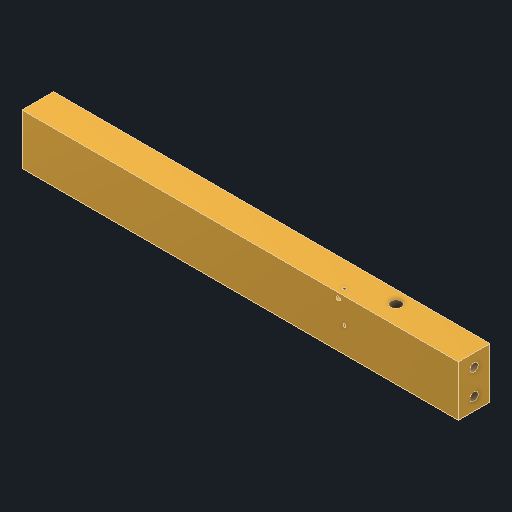
# Autodesk Inventor part: Main Piller
Saved by Autodesk Inventor 2027.1 (Build 311270010, 270A)
## iProperties
Created: 2025-09-16
Material: Brass, Soft Yellow
Document SubType Name: Modeling
Designer: SD
Density: 8.47 g/cm^3
Appearance: Brass - Satin
Mass: 2727.37 g
Surface Area: 492.65 cm^2
Volume: 340.921 cm^3
Project: Automatic Tea Steeping mechanism
Part Number: Main Piller
Thickness: 25.000 mm
Length: 345.000 mm
Width: 40.000 mm
BOM-Mass: 2.72737
BOM-Area: 0.049
Procurement: Fabricate - 1st round
Build Stage: 1
Preferred Material: C36000 Brass
Author: SD
Title: Main Piller
Autodesk Inventor part; units mm, degrees
ref_plane "YZ Plane" through (0, 0, 0) normal (1, 0, 0) x (0, 1, 0)
ref_plane "XZ Plane" through (0, 0, 0) normal (0, 1, 0) x (-1, 0, 0)
ref_plane "XY Plane" through (0, 0, 0) normal (0, 0, 1) x (1, 0, 0)
sketch "Sketch1" plane through (0, 0, 0) normal (1, 0, 0) x (0, 1, 0)
  line L0 (-20, 12.5) -> (20, 12.5)
  line L1 (20, 12.5) -> (20, -12.5)
  line L2 (20, -12.5) -> (-20, -12.5)
  line L3 (-20, -12.5) -> (-20, 12.5)
  line L4 (-20, 12.5) -> (20, -12.5) construction
  line L5 (20, 12.5) -> (-20, -12.5) construction
  point P0 (0, 0)
  dimension "Width" = 40
  dimension "Thickness" = 25
  constraints: 12 end point, 2 midpoint, 2 parallel, 1 horizontal, 1 perpendicular
  measures "Width" distance of L1.end L2.end
  measures "Thickness" distance of L0.end L1.end
extrude "Extrusion1" add sketch "Sketch1" along normal mid plane 345
sketch "Sketch2" plane through (-172.5, 0, 0) normal (-1, 0, 0) x (0, 0, 1)
  point P0 (0, 0)
  point P1 (0, 10)
  point P2 (0, -10)
  dimension "d4" = 20
  dimension "d5" = 10
  constraints: 2 vertical alignment
  measures "d4" distance of point (0, -10) point (0, 10)
  measures "d5" distance of point (0, 0) point (0, 10)
hole "Hole1" at (-172.5, 10, 0) at (-172.5, -10, 0) direction (1, 0, 0) diameter 4.917 depth 20 tip angle 118 thread size "M6x1" class "6H" standard "ISO Metric profile"
sketch "Sketch3" plane through (-172.5, 20, 12.5) normal (0, 1, 0) x (1, 0, 0)
  line L0 (345, 25) -> (345, 0) projected
  line L1 (0, 25) -> (345, 25) projected
  point P0 (172.5, 12.5)
  point P1 (280.7116, 15)
  dimension "d13" = 64.2884
  dimension "d14" = 10
  measures "d13" distance from line of point (280.712, 15) L0
  measures "d14" distance from line of point (280.712, 15) L1
hole "Hole2" at (108.2116, 20, -2.5) direction (0, -1, 0) diameter 8.376 depth 15 tip angle 118 thread size "M10x1.5" class "6H" standard "ISO Metric profile"
sketch "Sketch4" plane through (172.5, 20, -12.5) normal (0, 0, -1) x (-1, 0, 0)
  line L0 (345, 0) -> (345, -40) projected
  line L1 (0, -40) -> (345, -40) projected
  point P0 (172.5, -20)
  point P1 (325, -20)
  dimension "d22" = 20
  dimension "d23" = 20
  measures "d22" distance from line of point (325, -20) L0
  measures "d23" distance from line of point (325, -20) L1
hole "Hole3" at (-152.5, 0, -12.5) direction (0, 0, 1) diameter 8.376 depth 20 tip angle 118 thread size "M10x1.5" class "6H" standard "ISO Metric profile"
sketch "Sketch5" plane through (172.5, 0, 0) normal (1, 0, 0) x (0, 0, -1)
  circle A0 centre (0, 10) radius 2.4585 projected
  circle A1 centre (0, -10) radius 2.4585 projected
  point P0 (0, 0)
  constraints: 2 coincident
hole "Hole4" at (172.5, 10, 0) at (172.5, -10, 0) direction (-1, 0, 0) diameter 6.647 depth 16 tip angle 118 thread size "M8x1.25" class "6H" standard "ISO Metric profile"
sketch "Sketch6" plane through (-172.5, -20, 12.5) normal (0, 0, 1) x (1, 0, 0)
  line L0 (345, 40) -> (345, 0) projected
  point P0 (172.5, 20)
  point P1 (255, 20)
  dimension "d38" = 90
  constraints: 1 horizontal alignment
  measures "d38" distance from line of L0 point (255, 20)
hole "Hole5" at (82.5, 0, 12.5) direction (0, 0, -1) diameter 2.459 depth 10 tip angle 118 thread size "M3x0.5" class "6H" standard "ISO Metric profile"
sketch "Sketch7" plane through (-172.5, -20, 12.5) normal (0, 0, 1) x (1, 0, 0)
  line L0 (345, 40) -> (345, 0) projected
  line L1 (0, 40) -> (345, 40) projected
  point P0 (172.5, 20)
  point P1 (250, 36)
  dimension "d46" = 95
  dimension "d47" = 4
  measures "d46" distance from line of L0 point (250, 36)
  measures "d47" distance from line of L1 point (250, 36)
hole "Hole6" at (77.5, 16, 12.5) direction (0, 0, -1) diameter 3 depth 8
sketch "Sketch9" plane through (-172.5, -20, 12.5) normal (0, 0, 1) x (1, 0, 0)
  line L0 (251.5, 34.5) -> (248.5, 34.5)
  line L1 (248.5, 34.5) -> (248.5, 37.5)
  line L2 (248.5, 37.5) -> (251.5, 37.5)
  line L3 (251.5, 37.5) -> (251.5, 34.5)
  line L4 (251.5, 34.5) -> (248.5, 37.5) construction
  line L5 (248.5, 34.5) -> (251.5, 37.5) construction
  line L6 (0, 40) -> (345, 40) projected
  line L7 (345, 40) -> (345, 0) projected
  point P0 (250, 36)
  dimension "d67" = 4
  dimension "d68" = 95
  dimension "d69" = 3
  constraints: 12 end point, 2 midpoint, 2 parallel, 2 perpendicular, 1 horizontal
  measures "d67" distance from line of point (250, 36) L6
  measures "d68" distance from line of L7 point (250, 36)
  measures "d69" distance of L0.start L0.end
extrude "Extrusion2" [suppressed]
sketch "Sketch8" plane through (-172.5, 20, 12.5) normal (0, 1, 0) x (1, 0, 0)
  line L0 (345, 25) -> (345, 0) projected
  line L1 (0, 0) -> (345, 0) projected
  point P0 (172.5, 12.5)
  point P1 (250, 5)
  dimension "d55" = 95
  dimension "d56" = 5
  measures "d55" distance from line of L0 point (250, 5)
  measures "d56" distance from line of point (250, 5) L1
hole "Hole7" at (77.5, 20, 7.5) direction (0, -1, 0) diameter 2.459 depth 4 tip angle 118 thread size "M3x0.5" class "6H" standard "ISO Metric profile"
chamfer "Chamfer1" [suppressed]
chamfer "Chamfer2" distance 0.2 angle 45 1 edges at (77.5, 17.5, 12.5)
equation "\"d5\" = 0.5 * d4"
equation "\"d67\" = d47"
equation "\"d68\" = d46"
equation "\"d55\" = d46"
body "Solid1"
